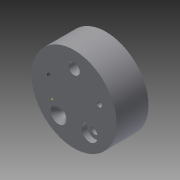
# Autodesk Inventor part: PartTL
Saved by Autodesk Inventor 2015 (Build 190159000, 159)
## iProperties
Created: 2015-01-30
Part Number: PartTL
Material: Generic
Document SubType Name: Modeling
Designer: PLTW-Stu-02
Density: 1 g/cm^3
Appearance: Default
Author: PLTW-Stu-02
Autodesk Inventor part; units mm, degrees
ref_plane "YZ Plane" through (0, 0, 0) normal (1, 0, 0) x (0, 1, 0)
ref_plane "XZ Plane" through (0, 0, 0) normal (0, 1, 0) x (-1, 0, 0)
ref_plane "XY Plane" through (0, 0, 0) normal (0, 0, 1) x (1, 0, 0)
sketch "Sketch1" plane through (0, 0, 0) normal (0, 0, 1) x (1, 0, 0)
  circle A0 centre (26.1399, 12.8792) radius 50.8
  point P0 (0, 0)
  dimension "d0" = 101.6
  constraints: 1 centre point
  measures "d0" diameter of A0
extrude "Extrusion1" add sketch "Sketch1" along normal blind 38.1
sketch "Sketch2" plane through (26.1399, 12.8792, 38.1) normal (0, 0, 1) x (1, 0, 0)
  point P0 (-26.1399, -12.8792)
sketch "Sketch3" plane through (26.1399, 12.8792, 38.1) normal (0, 0, 1) x (1, 0, 0)
  point P0 (-26.1399, -12.8792)
sketch "Sketch4" plane through (26.1399, 12.8792, 38.1) normal (0, 0, 1) x (1, 0, 0)
  circle A0 centre (0, 0) radius 31.6265 construction
  point P0 (-26.1399, -12.8792)
  point P1 (0, 31.6265)
  point P2 (-30.0786, 9.7731)
  point P3 (-18.5896, -25.5864)
  point P4 (18.5896, -25.5864)
  point P5 (30.0786, 9.7731)
  dimension "d5" = 360
  constraints: 1 vertical alignment, 8 other
hole "Hole1" at (56.2185, 22.6523, 38.1) direction (0, 0, -1) diameter 6.35 end through all
hole "Hole2" at (44.7295, -12.7072, 38.1) direction (0, 0, -1) diameter 9.525 end through all counterbore diameter 19.05 counterbore depth 6.35
hole "Hole3" at (7.5503, -12.7072, 38.1) direction (0, 0, -1) diameter 9.525 end through all countersink diameter 19.05 countersink angle 82
hole "Hole4" at (-3.9387, 22.6523, 38.1) direction (0, 0, -1) diameter 4.9784 end through all thread size "1/4-20 UNC" class "1B" standard "ANSI Unified Screw Threads"
hole "Hole5" at (26.1399, 44.5057, 38.1) direction (0, 0, -1) diameter 13.4874 end through all clearance for "Hex Head Bolt" size "1/2" standard "Ansi Unified Screw Threads"
body "Solid1"
